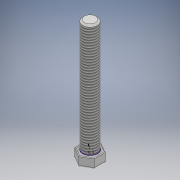
# Autodesk Inventor part: 零件3
Saved by Autodesk Inventor 2018 (Build 220112000, 112)
## iProperties
Created: 2023-04-30
Part Number: 零件3
Material: 常规
Document SubType Name: Sheet Metal
Designer: 47376
Density: 1 g/cm^3
Sheet Metal Rule: 默认_mm
Appearance: 默认
Author: 47376
Autodesk Inventor part; units mm, degrees
ref_plane "YZ Plane" through (0, 0, 0) normal (1, 0, 0) x (0, 1, 0)
ref_plane "XZ Plane" through (0, 0, 0) normal (0, 1, 0) x (-1, 0, 0)
ref_plane "XY Plane" through (0, 0, 0) normal (0, 0, 1) x (1, 0, 0)
sketch "草图1" plane through (0, 0, 0) normal (0, 0, 1) x (1, 0, 0)
  circle A0 centre (0, 0) radius 2.25
  dimension "d0" = 4.5
  constraints: 1 centre point, 1 coincident
  measures "d0" diameter of A0
extrude "拉伸1" add sketch "草图1" along normal blind 35
thread "螺纹1" size "M4.5x0.75" class "6g" standard "ANSI Metric M Profile" full length
sketch "草图4" plane through (0, 0, 0) normal (0, 0, -1) x (-1, 0, 0)
  line L0 (0, -3.5) -> (-3.0311, -1.75)
  line L1 (-3.0311, -1.75) -> (-3.0311, 1.75)
  line L2 (-3.0311, 1.75) -> (0, 3.5)
  line L3 (0, 3.5) -> (3.0311, 1.75)
  line L4 (3.0311, 1.75) -> (3.0311, -1.75)
  line L5 (3.0311, -1.75) -> (0, -3.5)
  point P0 (0, 0)
  point P1 (0, 0)
  constraints: 12 end point, 13 other
sketch "草图5" plane through (0, 0, 0) normal (0, 0, -1) x (-1, 0, 0)
  point P0 (0, 0)
extrude "拉伸4" add sketch "草图4" along normal blind 3
fillet "圆角3" radius 0.5 6 edges at (-1.5155, -2.625, -3) (-3.0311, 0, -3) (-1.5155, 2.625, -3) (1.5155, 2.625, -3) (3.0311, 0, -3) (1.5155, -2.625, -3)
fillet "圆角4" radius 0.2 6 edges at (1.5155, -2.625, 0) (3.0311, 0, 0) (1.5155, 2.625, 0) (-1.5155, -2.625, 0) (-1.5155, 2.625, 0) (-3.0311, 0, 0)
sketch "草图6" plane through (0, 0, -3) normal (0, 0, -1) x (-1, 0, 0)
  circle A0 centre (0, 0) radius 1.5
  dimension "d20" = 3
  constraints: 1 centre point, 1 coincident
  measures "d20" diameter of A0
extrude "拉伸5" cut sketch "草图6" against normal blind 2
chamfer "倒角1" distance 0.5 angle 45 1 edges at (-2.25, 0, 35)
equation "\"折弯半径\" = 厚度"
equation "\"折弯释压宽度\" = 厚度"
equation "\"折弯释压深度\" = 0.5 * 厚度"
equation "\"拐角释压尺寸\" = 4 * 厚度"
equation "\"最小余量\" = 2 * 厚度"
equation "\"过渡半径\" = 折弯半径"
equation "\"Jacobi半径尺寸\" = 折弯半径"
equation "\"间隙大小\" = 厚度"
equation "\"厚度\" = 0.5"
